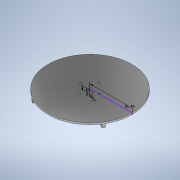
# Autodesk Inventor part: motor platform reaction wheel
Saved by Autodesk Inventor 2022 (Build 260153000, 153)
## iProperties
Created: 2021-07-29
Part Number: motor platform reaction wheel
Material: ABS Plastic
Document SubType Name: Modeling
Designer: samlo
Density: 1.06 g/cm^3
Appearance: Honed
Author: samlo
Autodesk Inventor part; units mm, degrees
ref_plane "YZ Plane" through (0, 0, 0) normal (1, 0, 0) x (0, 1, 0)
ref_plane "XZ Plane" through (0, 0, 0) normal (0, 1, 0) x (-1, 0, 0)
ref_plane "XY Plane" through (0, 0, 0) normal (0, 0, 1) x (1, 0, 0)
sketch "Sketch1" plane through (0, 0, 0) normal (0, 0, 1) x (1, 0, 0)
  line L0 (4, 0) -> (6, 0)
  line L1 (6, 0) -> (6, 6)
  line L2 (6, 6) -> (76.45, 6)
  line L3 (76.45, 6) -> (76.45, 9)
  line L4 (4, 6) -> (4, 0)
  line L5 (0, 9) -> (0, 6)
  line L6 (0, 6) -> (4, 6)
  line L7 (0, 9) -> (13.95, 9)
  line L8 (16.45, 9) -> (76.45, 9)
  line L9 (13.95, 9) -> (16.45, 9)
  point P0 (0, 0)
  dimension "d0" = 4
  dimension "d1" = 6
  dimension "d2" = 0
  dimension "d3" = 3
  dimension "d4" = 2
  dimension "d39" = 76.45
  constraints: 20 end point, 4 perpendicular, 3 horizontal, 2 point on line
  measures "d0" distance of L5.end L4.start
  measures "d1" distance of L4.start L0.start
  measures "d2" distance from line of point (0, 0) L0
  measures "d3" distance of L5.start L5.end
  measures "d4" distance of L0.start L0.end
  measures "d39" distance of L3.end L5.start
revolve "Revolution1" add sketch "Sketch1" angle 360 about axis through (0, 9, 0) along (0, -1, 0)
thread "Thread1" size "M8x1.25" class "6H" standard "ANSI Metric M Profile" full length
sketch "Sketch5" plane through (0, 6, 0) normal (0, -1, 0) x (1, 0, 0)
  circle A0 centre (0, 0) radius 76.45 projected
  circle A1 centre (0, 0) radius 6 projected
  circle A2 centre (0, 0) radius 4 projected
  line L0 (-5.1962, -3) -> (-66.2076, -38.225)
  line L1 (-63.7866, -42.1411) -> (-1.873, -5.7002)
  line L2 (42.1411, -63.7866) -> (5.7002, -1.873)
  line L3 (3, -5.1962) -> (38.225, -66.2076)
  line L4 (63.7866, 42.1411) -> (1.873, 5.7002)
  line L5 (5.1962, 3) -> (66.2076, 38.225)
  line L6 (-42.1411, 63.7866) -> (-5.7002, 1.873)
  line L7 (-3, 5.1962) -> (-38.225, 66.2076)
  arc A3 (38.225, -66.2076) -> (42.1411, -63.7866) centre (0, 0) ccw
  arc A4 (66.2076, 38.225) -> (63.7866, 42.1411) centre (0, 0) ccw
  arc A5 (-38.225, 66.2076) -> (-42.1411, 63.7866) centre (0, 0) ccw
  arc A6 (-66.2076, -38.225) -> (-63.7866, -42.1411) centre (0, 0) ccw
  arc A7 (-5.1962, -3) -> (-1.873, -5.7002) centre (0, 0) ccw
  arc A8 (-3, 5.1962) -> (-5.7002, 1.873) centre (0, 0) ccw
  arc A9 (3, -5.1962) -> (5.7002, -1.873) centre (0, 0) ccw
  arc A10 (5.1962, 3) -> (1.873, 5.7002) centre (0, 0) ccw
  point P0 (0, 0)
  point P1 (-38.225, 66.2076)
  point P2 (-42.1411, 63.7866)
  point P3 (-5.7002, 1.873)
  point P4 (5.1962, 3)
  point P5 (66.2076, 38.225)
  point P6 (63.7866, 42.1411)
  point P7 (1.873, 5.7002)
  point P8 (38.225, -66.2076)
  point P9 (42.1411, -63.7866)
  point P10 (5.7002, -1.873)
  dimension "d35" = 360
  constraints: 20 point on circle, 16 end point, 8 centre point, 2 coincident, 25 other
extrude "Extrusion3" add sketch "Sketch5" along normal blind 6 contours L5 A1 L4 A0 | A0 L3 A1 L2 | L7 A1 L6 A0 | A0 L0 A1 L1
sketch "Sketch6" plane through (0, 9, 0) normal (0, 1, 0) x (1, 0, 0)
  circle A0 centre (0, 0) radius 20.5
  circle A1 centre (0, 0) radius 16.9
  circle A2 centre (0, 16.9) radius 1.6
  circle A3 centre (-16.9, 0) radius 1.6
  circle A4 centre (0, -16.9) radius 1.6
  circle A5 centre (16.9, 0) radius 1.6
  dimension "d41" = 33.8
  dimension "d40" = 41
  dimension "d42" = 3.2
  dimension "d45" = 360
  constraints: 5 centre point, 2 coincident, 1 vertical alignment, 11 other
  measures "d40" diameter of A0
  measures "d42" diameter of A2
extrude "Extrusion4" cut sketch "Sketch6" against normal blind 10 contours A1 A5 | A1 A5 | A2 A1 | A1 A2 | A4 A1 | A1 A4 | A3 A1 | A1 A3
body "Solid1"
